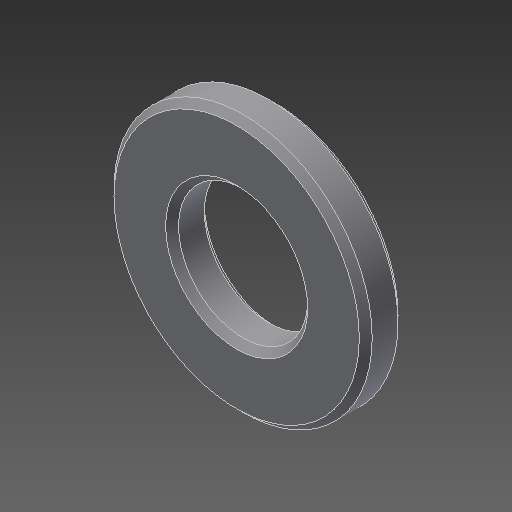
# Autodesk Inventor part: WSSM20-10-3
Saved by Autodesk Inventor 2021.1 (Build 251245010, 245A)
## iProperties
Created: 2008-11-14
Part Number: WSSM20-10-3
Material: MISUMI
Document SubType Name: Modeling
Density: 1 g/cm^3
Mass: 0.683296 g
Surface Area: 6.98773 cm^2
Volume: 0.683296 cm^3
Appearance: 既定
Title: 金属ワッシャ
Autodesk Inventor part; units mm, degrees
ref_plane "YZ Plane" through (0, 0, 0) normal (1, 0, 0) x (0, 1, 0)
ref_plane "XZ Plane" through (0, 0, 0) normal (0, 1, 0) x (-1, 0, 0)
ref_plane "XY Plane" through (0, 0, 0) normal (0, 0, 1) x (1, 0, 0)
sketch "スケッチ1" plane through (0, 0, 0) normal (0, 0, 1) x (1, 0, 0)
  circle A0 centre (0, 0) radius 10
  dimension "d0" = 20
  constraints: 1 centre point, 1 coincident
  measures "d0" diameter of A0
extrude "押し出し1" add sketch "スケッチ1" along normal blind 3
sketch "スケッチ2" plane through (0, 0, 3) normal (0, 0, 1) x (1, 0, 0)
  circle A0 centre (0, 0) radius 10 projected
hole "穴1" at (0, 0, 3) direction (0, 0, -1) diameter 10 end through all
chamfer "面取り1" distance 0.5 angle 45 4 edges at (-10, 0, 3) (-10, 0, 0) (0, 5, 3) (0, 5, 0)
